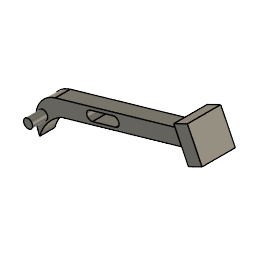
Arm button (Autodesk Fusion 360 design; units mm, degrees)
part number: 2026-06-02-14-34-20-649
Autodesk Fusion 360 part; units mm, degrees
sketch "arm button" plane through (0, 0, 0) normal (0, 1, 0) x (1, 0, 0)
  circle A0 centre (0, 0) radius 6.5 construction
  circle A1 centre (0, 0) radius 7.75 construction
  line L0 (0, 0) -> (1.3458, -7.6323) construction
  line L1 (0, 0) -> (-2.8494, -5.8422) construction
  arc A2 (-2.8494, -5.8422) -> (1.3458, -7.6323) centre (0.5379, -3.7147) ccw construction
  line L2 (0, 0) -> (7.75, 0) construction
  line L3 (1.3458, -7.6323) -> (3.109, -17.6323) construction
  circle A3 centre (2.9976, -17) radius 2.5 construction
  line L4 (-2.8494, -5.8422) -> (-3.5774, -7.8422)
  arc A4 (-3.5774, -7.8422) -> (2.3063, -19.4025) centre (4.7595, -10.8765) ccw
  arc A5 (-2.8494, -5.8422) -> (4.2238, -14.8214) centre (11.5816, -1.7499) ccw
  line L5 (-2.8494, -5.8422) -> (-1.0861, -15.8422) construction
  line L6 (2.3063, -19.4025) -> (45.6474, -31.8735)
  line L7 (4.2238, -14.8214) -> (47.8427, -27.3723)
  line L8 (47.8427, -27.3723) -> (45.6474, -31.8735)
  circle A6 centre (-1.6566, -12.607) radius 1.5
  line L9 (14.5654, -18.7677) -> (22.2534, -20.9798)
  line L10 (13.7358, -21.6507) -> (21.4239, -23.8628)
  arc A7 (21.4239, -23.8628) -> (22.2534, -20.9798) centre (21.8387, -22.4213) ccw
  arc A8 (14.5654, -18.7677) -> (13.7358, -21.6507) centre (14.1506, -20.2092) ccw
  dimension "d1" = 13
  dimension "d2" = 15.5
  dimension "d3" = 36
  dimension "d5" = 80
  dimension "d6" = 4
  dimension "d7" = 5
  dimension "d9" = 2
  dimension "d10" = 30
  dimension "d11" = 17
  dimension "d12" = 15
  dimension "d13" = 55
  dimension "d15" = 10
  dimension "d16" = 10
  dimension "d22" = 3
  dimension "d28" = 6.4
  dimension "d29" = 3
  dimension "d30" = 3
  dimension "d31" = 17
  dimension "d32" = 8
  dimension "d33" = 2.5
  constraint coincident A0.centre A1.centre
  constraint concentric A0 A1
  constraint coincident A1 L0.end
  constraint coincident A0 L1.end
  constraint coincident A1 L2.end
  constraint horizontal L2
  constraint parallel L0 L3
  constraint coincident L3 A3.centre
  constraint tangent L4 A4
  constraint coincident A3 A4.end
  constraint coincident A3 A5.end
  constraint tangent A3 A5
  constraint tangent A3 A4
  constraint parallel L3 L5
  constraint tangent A3 L6
  constraint parallel L6 L7
  constraint parallel L1 L8
  constraint coincident L5 A6.centre
  constraint tangent L9 A7
  constraint tangent L10 A7
  constraint tangent L10 A8
  constraint tangent L9 A8
  constraint parallel L6 L10
  measures "d1" diameter of A0
  measures "d2" diameter of A1
  measures "d3" angle of L0 L1
  measures "d5" angle of L0 L2
  measures "d6" radius of A2
  measures "d7" diameter of A3
  measures "d9" vertical distance of L1.end L4.end
  measures "d10" angle of L4 L5
  measures "d11" vertical distance of A0.centre A3.centre
  measures "d12" radius of A5
  measures "d13" distance of L1 L7.end
  measures "d15" vertical distance of L1.end L5.end
  measures "d16" vertical distance of L0.end L3.end
  measures "d22" diameter of A6
  measures "d28" distance of A3.centre A6.centre
  measures "d29" diameter of A8
  measures "d30" diameter of A7
  measures "d31" horizontal distance of L1.end A8.centre
  measures "d32" distance of A8.centre A7.centre
  measures "d33" distance of L6 A7.centre
extrude "Extrude1" add sketch "arm button" against normal blind 5 contours L4 A4 A5 L6 L7 L8 | A6 | L9 L10 A7 A8
sketch "button" plane through (49.4337, 0, 24.1104) normal (0.898794, 0, 0.438371) x (0, 1, 0)
  line L0 (0, 3.6292) -> (0, 8.6372)
  line L1 (0, 8.6372) -> (-5, 8.6372)
  line L2 (-5, 8.6372) -> (-5, 3.6292)
  line L3 (-5, 3.6292) -> (0, 3.6292)
  line L4 (-5, 3.6292) -> (-5, 8.6372)
  line L5 (0, 8.6372) -> (-5, 8.6372)
  line L6 (0, 3.6292) -> (0, 8.6372)
  line L7 (0, 3.6292) -> (-5, 3.6292)
  line L8 (-8, 0.6292) -> (3, 0.6292)
  line L9 (3, 0.6292) -> (3, 11.6372)
  line L10 (3, 11.6372) -> (-8, 11.6372)
  line L11 (-8, 11.6372) -> (-8, 0.6292)
  dimension "d19" = 3
extrude "Extrude2" add sketch "button" along normal blind 5 contours L0 L1 L2 L3 L4 L5 L6 L7 | L8 L9 L10 L11
extrude "Extrude3" add sketch "arm button" against normal blind 10 contours A6
extrude "Extrude4" cut sketch "arm button" against normal up to surface (5 mm away) contours L9 L10 A7 A8
named bodies: "Arm button"
